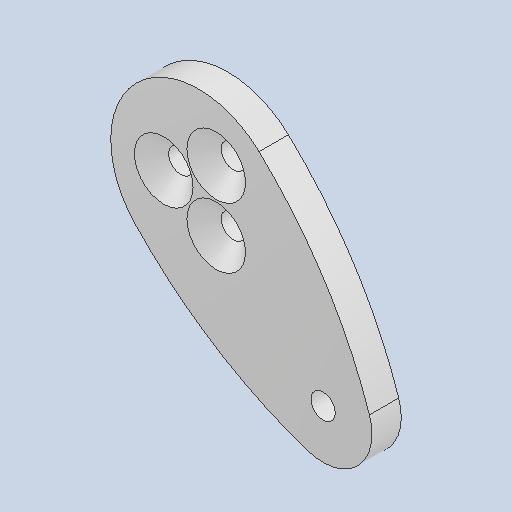
# Autodesk Inventor part: クランク_前
Saved by Autodesk Inventor 2022.2 (Build 262287000, 287)
## iProperties
Created: 2022-01-08
Part Number: クランク_前
Material: Aluminum 2014-T6
Document SubType Name: Modeling
Designer: acps
Density: 2.78927 g/cm^3
Appearance: Satin
Author: acps
Autodesk Inventor part; units mm, degrees
ref_plane "YZ Plane" through (0, 0, 0) normal (1, 0, 0) x (0, 1, 0)
ref_plane "XZ Plane" through (0, 0, 0) normal (0, 1, 0) x (-1, 0, 0)
ref_plane "XY Plane" through (0, 0, 0) normal (0, 0, 1) x (1, 0, 0)
sketch "Sketch1" plane through (0, 0, 0) normal (0, 0, 1) x (1, 0, 0)
  line L0 (0.1155, 0) -> (-12.6125, 12.7279) construction
  line L1 (0.1155, 0) -> (18.1155, 0) construction
  circle A0 centre (0.1155, 0) radius 1.25
  line L2 (-12.6125, 12.7279) -> (0.1155, 0) construction
  line L3 (-16.148, 9.1924) -> (-3.4778, -3.4778) construction
  line L4 (3.5933, 3.5933) -> (-9.0769, 16.2635) construction
  arc A1 (-9.0769, 16.2635) -> (-16.148, 9.1924) centre (-12.6125, 12.7279) ccw construction
  arc A2 (-1.4689, -4.7423) -> (4.8578, 1.5844) centre (0.1155, 0) ccw
  circle A3 centre (-10.8227, 15.8279) radius 1.25
  circle A4 centre (-10.8227, 15.8279) radius 3.1 construction
  circle A5 centre (-16.192, 12.7279) radius 3.1 construction
  circle A6 centre (-16.192, 12.7279) radius 1.25
  circle A7 centre (-10.8227, 9.6279) radius 3.1 construction
  circle A8 centre (-10.8227, 9.6279) radius 1.25
  circle A9 centre (-12.6125, 12.7279) radius 9
  arc A10 (-19.1549, 6.5476) -> (-1.4689, -4.7423) centre (12.1976, 36.1644) ccw
  line L5 (-11.009, -0.1893) -> (-5.3521, 5.4676) construction
  arc A11 (4.8578, 1.5844) -> (-6.4322, 19.2704) centre (-36.0489, -12.0821) ccw
  point P0 (0, 0)
  point P1 (-6.2485, 6.364)
  point P2 (-6.4322, 19.2704)
  dimension "d9" = 18
  dimension "d2" = 18
  dimension "d3" = 135
  dimension "d4" = 2.5
  dimension "d5" = 5
  dimension "d6" = 2.5
  dimension "d7" = 6.2
  dimension "d8" = 360
  dimension "d10" = 8
  constraints: 14 end point, 11 centre point, 9 point on circle, 6 coincident, 5 tangent, 3 equal length, 3 symmetric about line, 1 equal radius, 1 horizontal, 1 midpoint, 1 perpendicular, 1 point on line, 1 vertical alignment, 19 other
  measures "d2" distance of L0.start L0.end
  measures "d3" angle of L1 L0
  measures "d4" diameter of A0
  measures "d5" radius of A2
  measures "d6" diameter of A3
  measures "d7" diameter of A4
  measures "d10" distance of L5.start L5.end
extrude "Extrusion1" add sketch "Sketch1" along normal blind 3
chamfer "Chamfer1" distance 1.75 angle 45 3 edges at (-12.0727, 15.8279, 3) (-17.442, 12.7279, 3) (-12.0727, 9.6279, 3)
body "Solid1"
